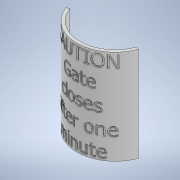
# Autodesk Inventor part: warningSignV1
Saved by Autodesk Inventor 2021.2 (Build 252289000, 289)
## iProperties
Created: 2020-11-24
Part Number: warningSignV1
Material: Generic
Document SubType Name: Modeling
Designer: robst
Density: 1 g/cm^3
Appearance: Default
Author: robst
Autodesk Inventor part; units mm, degrees
ref_plane "YZ Plane" through (0, 0, 0) normal (1, 0, 0) x (0, 1, 0)
ref_plane "XZ Plane" through (0, 0, 0) normal (0, 1, 0) x (-1, 0, 0)
sketch "Sketch1" plane through (0, 0, 0) normal (0, 1, 0) x (-1, 0, 0)
  arc A0 (65.9911, 38.1) -> (-65.4234, 39.0668) centre (0, 0) ccw
  arc A1 (72.6124, 39.2675) -> (-71.4904, 41.275) centre (0, 0) ccw
  line L0 (0, 0) -> (0, -82.55) construction
  arc A2 (71.6046, 26.0619) -> (-71.6046, 26.0619) centre (0, 0) ccw
  arc A3 (77.5716, 28.2338) -> (-77.5716, 28.2338) centre (0, 0) ccw
  line L1 (0, 0) -> (77.5716, 28.2338) construction
  line L2 (0, 0) -> (-77.5716, 28.2338) construction
  line L3 (-77.5716, 28.2338) -> (-71.6046, 26.0619)
  line L4 (77.5716, 28.2338) -> (71.6046, 26.0619)
  point P0 (-65.4234, 39.0668)
  point P1 (65.9911, 38.1)
  point P2 (72.6124, 39.2675)
  point P3 (-71.4904, 41.275)
  dimension "d0" = 152.4
  dimension "d9" = 6.35
  dimension "d10" = 110
  dimension "d11" = 110
  constraints: 10 end point, 8 point on circle, 4 centre point, 4 coincident, 2 concentric, 2 point on line, 1 vertical
  measures "d0" diameter of A0
  measures "d9" radial gap between concentric circles of A1 A0
  measures "d10" angle of L1 L0
  measures "d11" angle of L2 L0
extrude "Extrusion1" add sketch "Sketch1" along normal blind 203.2
ref_plane "Work Plane1" through (0, 0, 82.55) normal (0, 0, 1) x (1, 0, 0)
sketch "Sketch3" plane through (0, 0, 82.55) normal (0, 0, 1) x (1, 0, 0)
  line L0 (-72.043, 0) -> (-72.043, 203.2) projected
  line L1 (71.4904, 0) -> (71.4904, 203.2) projected
  line L2 (77.5716, 203.2) -> (-77.5716, 203.2) projected
  line L3 (77.5716, 0) -> (-77.5716, 0) projected
  line L4 (-72.043, 177.8) -> (71.4904, 177.8) construction
  spline S0 degree 2 poles (-60.9358, 172.2672) (-63.4058, 172.2672) (-67.5842, 173.9344) (-69.1074, 175.6017) knots 0 0 0 1 2 2 2
  spline S1 degree 2 poles (-69.1074, 175.6017) (-70.6306, 177.2484) (-72.2979, 182.1884) (-72.2979, 185.3994) knots 0 0 0 1 2 2 2
  spline S2 degree 2 poles (-72.2979, 185.3994) (-72.2979, 188.5899) (-70.6718, 193.3241) (-69.128, 195.0736) knots 0 0 0 1 2 2 2
  spline S3 degree 2 poles (-69.128, 195.0736) (-67.6048, 196.7821) (-63.447, 198.5728) (-60.874, 198.5728) knots 0 0 0 1 2 2 2
  spline S4 degree 2 poles (-60.874, 198.5728) (-59.5979, 198.5728) (-57.3543, 198.2023) (-56.4074, 197.9142) knots 0 0 0 1 2 2 2
  spline S5 degree 2 poles (-56.4074, 197.9142) (-55.5841, 197.6466) (-53.8757, 196.885) (-53.0317, 196.4322) knots 0 0 0 1 2 2 2
  line L5 (-53.0317, 196.4322) -> (-53.0317, 192.3566)
  line L6 (-53.0317, 192.3566) -> (-53.2993, 192.3566)
  spline S6 degree 2 poles (-53.2993, 192.3566) (-53.7522, 192.7683) (-55.1518, 193.921) (-56.1604, 194.4767) knots 0 0 0 1 2 2 2
  spline S7 degree 2 poles (-56.1604, 194.4767) (-57.1278, 195.0119) (-59.4126, 195.6912) (-60.8946, 195.6912) knots 0 0 0 1 2 2 2
  spline S8 degree 2 poles (-60.8946, 195.6912) (-62.5207, 195.6912) (-65.423, 194.3532) (-66.5139, 193.077) knots 0 0 0 1 2 2 2
  spline S9 degree 2 poles (-66.5139, 193.077) (-67.5842, 191.7803) (-68.7781, 187.8488) (-68.7781, 185.3994) knots 0 0 0 1 2 2 2
  spline S10 degree 2 poles (-68.7781, 185.3994) (-68.7781, 182.7853) (-67.5225, 179.0185) (-66.4316, 177.7218) knots 0 0 0 1 2 2 2
  spline S11 degree 2 poles (-66.4316, 177.7218) (-65.3612, 176.4662) (-62.5001, 175.19) (-60.8946, 175.19) knots 0 0 0 1 2 2 2
  spline S12 degree 2 poles (-60.8946, 175.19) (-59.4332, 175.19) (-56.9426, 175.9104) (-55.9752, 176.4456) knots 0 0 0 1 2 2 2
  spline S13 degree 2 poles (-55.9752, 176.4456) (-55.0489, 176.9808) (-53.6698, 178.0923) (-53.2787, 178.4834) knots 0 0 0 1 2 2 2
  line L7 (-53.2787, 178.4834) -> (-53.0317, 178.4834)
  line L8 (-53.0317, 178.4834) -> (-53.0317, 174.449)
  spline S14 degree 2 poles (-53.0317, 174.449) (-53.8757, 174.0579) (-55.3577, 173.3375) (-56.4074, 173.0082) knots 0 0 0 1 2 2 2
  spline S15 degree 2 poles (-56.4074, 173.0082) (-57.5189, 172.6377) (-59.4126, 172.2672) (-60.9358, 172.2672) knots 0 0 0 1 2 2 2
  line L9 (-52.6201, 172.72) -> (-44.0573, 198.12)
  line L10 (-44.0573, 198.12) -> (-39.8995, 198.12)
  line L11 (-39.8995, 198.12) -> (-31.3368, 172.72)
  line L12 (-31.3368, 172.72) -> (-34.8977, 172.72)
  line L13 (-34.8977, 172.72) -> (-37.203, 179.8213)
  line L14 (-37.203, 179.8213) -> (-46.8979, 179.8213)
  line L15 (-46.8979, 179.8213) -> (-49.2032, 172.72)
  line L16 (-49.2032, 172.72) -> (-52.6201, 172.72)
  line L17 (-38.1293, 182.703) -> (-42.0607, 194.662)
  line L18 (-42.0607, 194.662) -> (-45.9716, 182.703)
  line L19 (-45.9716, 182.703) -> (-38.1293, 182.703)
  spline S16 degree 2 poles (-19.7277, 172.1848) (-21.9713, 172.1848) (-25.3058, 173.3581) (-26.4791, 174.5313) knots 0 0 0 1 2 2 2
  spline S17 degree 2 poles (-26.4791, 174.5313) (-27.817, 175.8487) (-28.9079, 179.5537) (-28.9079, 182.2707) knots 0 0 0 1 2 2 2
  line L20 (-28.9079, 182.2707) -> (-28.9079, 198.12)
  line L21 (-28.9079, 198.12) -> (-25.5322, 198.12)
  line L22 (-25.5322, 198.12) -> (-25.5322, 182.2707)
  spline S18 degree 2 poles (-25.5322, 182.2707) (-25.5322, 180.5006) (-25.0794, 178.1129) (-24.4413, 177.1454) knots 0 0 0 1 2 2 2
  spline S19 degree 2 poles (-24.4413, 177.1454) (-23.762, 176.1163) (-21.4155, 175.0665) (-19.7277, 175.0665) knots 0 0 0 1 2 2 2
  spline S20 degree 2 poles (-19.7277, 175.0665) (-18.1428, 175.0665) (-15.6727, 176.1163) (-14.9935, 177.1454) knots 0 0 0 1 2 2 2
  spline S21 degree 2 poles (-14.9935, 177.1454) (-14.3554, 178.1129) (-13.9026, 180.48) (-13.9026, 182.1884) knots 0 0 0 1 2 2 2
  line L23 (-13.9026, 182.1884) -> (-13.9026, 198.12)
  line L24 (-13.9026, 198.12) -> (-10.5269, 198.12)
  line L25 (-10.5269, 198.12) -> (-10.5269, 182.2707)
  spline S22 degree 2 poles (-10.5269, 182.2707) (-10.5269, 179.6155) (-11.5972, 175.8281) (-12.9557, 174.5313) knots 0 0 0 1 2 2 2
  spline S23 degree 2 poles (-12.9557, 174.5313) (-14.1701, 173.3375) (-17.3812, 172.1848) (-19.7277, 172.1848) knots 0 0 0 1 2 2 2
  line L26 (0.2383, 172.72) -> (0.2383, 195.1148)
  line L27 (0.2383, 195.1148) -> (-8.2833, 195.1148)
  line L28 (-8.2833, 195.1148) -> (-8.2833, 198.12)
  line L29 (-8.2833, 198.12) -> (12.1355, 198.12)
  line L30 (12.1355, 198.12) -> (12.1355, 195.1148)
  line L31 (12.1355, 195.1148) -> (3.614, 195.1148)
  line L32 (3.614, 195.1148) -> (3.614, 172.72)
  line L33 (3.614, 172.72) -> (0.2383, 172.72)
  line L34 (23.5799, 172.72) -> (13.741, 172.72)
  line L35 (13.741, 172.72) -> (13.741, 175.3135)
  line L36 (13.741, 175.3135) -> (16.9726, 175.3135)
  line L37 (16.9726, 175.3135) -> (16.9726, 195.5265)
  line L38 (16.9726, 195.5265) -> (13.741, 195.5265)
  line L39 (13.741, 195.5265) -> (13.741, 198.12)
  line L40 (13.741, 198.12) -> (23.5799, 198.12)
  line L41 (23.5799, 198.12) -> (23.5799, 195.5265)
  line L42 (23.5799, 195.5265) -> (20.3483, 195.5265)
  line L43 (20.3483, 195.5265) -> (20.3483, 175.3135)
  line L44 (20.3483, 175.3135) -> (23.5799, 175.3135)
  line L45 (23.5799, 175.3135) -> (23.5799, 172.72)
  spline S24 degree 2 poles (45.7277, 195.2177) (47.1686, 193.5299) (48.7741, 188.5899) (48.7741, 185.42) knots 0 0 0 1 2 2 2
  spline S25 degree 2 poles (48.7741, 185.42) (48.7741, 182.3325) (47.2098, 177.3307) (45.7277, 175.6429) knots 0 0 0 1 2 2 2
  spline S26 degree 2 poles (45.7277, 175.6429) (44.1634, 173.8727) (40.0261, 172.1848) (37.5355, 172.1848) knots 0 0 0 1 2 2 2
  spline S27 degree 2 poles (37.5355, 172.1848) (34.9626, 172.1848) (30.8459, 173.9344) (29.3433, 175.6429) knots 0 0 0 1 2 2 2
  spline S28 degree 2 poles (29.3433, 175.6429) (27.8819, 177.3307) (26.3175, 182.2913) (26.3175, 185.42) knots 0 0 0 1 2 2 2
  spline S29 degree 2 poles (26.3175, 185.42) (26.3175, 188.6104) (27.9025, 193.4681) (29.3639, 195.2177) knots 0 0 0 1 2 2 2
  spline S30 degree 2 poles (29.3639, 195.2177) (30.8459, 196.9056) (34.9832, 198.6552) (37.5355, 198.6552) knots 0 0 0 1 2 2 2
  spline S31 degree 2 poles (37.5355, 198.6552) (40.129, 198.6552) (44.2869, 196.8438) (45.7277, 195.2177) knots 0 0 0 1 2 2 2
  spline S32 degree 2 poles (45.2543, 185.42) (45.2543, 187.9312) (44.1634, 191.8215) (43.1754, 193.0976) knots 0 0 0 1 2 2 2
  spline S33 degree 2 poles (43.1754, 193.0976) (42.1668, 194.415) (39.3263, 195.7323) (37.5561, 195.7323) knots 0 0 0 1 2 2 2
  spline S34 degree 2 poles (37.5561, 195.7323) (35.7242, 195.7323) (32.966, 194.4561) (31.9162, 193.0976) knots 0 0 0 1 2 2 2
  spline S35 degree 2 poles (31.9162, 193.0976) (30.9076, 191.8009) (29.8373, 187.89) (29.8373, 185.42) knots 0 0 0 1 2 2 2
  spline S36 degree 2 poles (29.8373, 185.42) (29.8373, 180.4182) (34.0363, 175.1077) (37.5561, 175.1077) knots 0 0 0 1 2 2 2
  spline S37 degree 2 poles (37.5561, 175.1077) (41.0759, 175.1077) (45.2543, 180.4182) (45.2543, 185.42) knots 0 0 0 1 2 2 2
  line L46 (70.6543, 172.72) -> (66.867, 172.72)
  line L47 (66.867, 172.72) -> (55.6284, 194.6208)
  line L48 (55.6284, 194.6208) -> (55.6284, 172.72)
  line L49 (55.6284, 172.72) -> (52.4791, 172.72)
  line L50 (52.4791, 172.72) -> (52.4791, 198.12)
  line L51 (52.4791, 198.12) -> (57.2751, 198.12)
  line L52 (57.2751, 198.12) -> (67.5051, 178.01)
  line L53 (67.5051, 178.01) -> (67.5051, 198.12)
  line L54 (67.5051, 198.12) -> (70.6543, 198.12)
  line L55 (70.6543, 198.12) -> (70.6543, 172.72)
  spline S38 degree 2 poles (-22.9284, 130.3638) (-25.6248, 130.3638) (-30.0915, 132.0105) (-31.697, 133.6777) knots 0 0 0 1 2 2 2
  spline S39 degree 2 poles (-31.697, 133.6777) (-33.3025, 135.3656) (-35.0109, 140.3468) (-35.0109, 143.5784) knots 0 0 0 1 2 2 2
  spline S40 degree 2 poles (-35.0109, 143.5784) (-35.0109, 146.6453) (-33.2819, 151.503) (-31.6764, 153.232) knots 0 0 0 1 2 2 2
  spline S41 degree 2 poles (-31.6764, 153.232) (-30.1326, 154.8993) (-25.6043, 156.7106) (-22.9078, 156.7106) knots 0 0 0 1 2 2 2
  spline S42 degree 2 poles (-22.9078, 156.7106) (-21.6111, 156.7106) (-19.2646, 156.3401) (-18.1942, 156.0108) knots 0 0 0 1 2 2 2
  spline S43 degree 2 poles (-18.1942, 156.0108) (-17.3297, 155.7638) (-15.2302, 154.8581) (-14.5921, 154.5288) knots 0 0 0 1 2 2 2
  line L56 (-14.5921, 154.5288) -> (-14.5921, 150.4533)
  line L57 (-14.5921, 150.4533) -> (-14.8803, 150.4533)
  spline S44 degree 2 poles (-14.8803, 150.4533) (-15.5184, 151.009) (-16.8563, 152.0176) (-18.0913, 152.594) knots 0 0 0 1 2 2 2
  spline S45 degree 2 poles (-18.0913, 152.594) (-19.1205, 153.1085) (-21.7757, 153.7878) (-23.2989, 153.7878) knots 0 0 0 1 2 2 2
  spline S46 degree 2 poles (-23.2989, 153.7878) (-26.9628, 153.7878) (-31.4911, 148.2714) (-31.4911, 143.6813) knots 0 0 0 1 2 2 2
  spline S47 degree 2 poles (-31.4911, 143.6813) (-31.4911, 141.129) (-30.2973, 137.3004) (-29.1652, 135.9831) knots 0 0 0 1 2 2 2
  spline S48 degree 2 poles (-29.1652, 135.9831) (-28.0743, 134.6658) (-24.9868, 133.2867) (-23.0519, 133.2867) knots 0 0 0 1 2 2 2
  spline S49 degree 2 poles (-23.0519, 133.2867) (-21.6317, 133.2867) (-18.7911, 133.6983) (-17.8237, 134.11) knots 0 0 0 1 2 2 2
  line L58 (-17.8237, 134.11) -> (-17.8237, 140.6761)
  line L59 (-17.8237, 140.6761) -> (-23.7106, 140.6761)
  line L60 (-23.7106, 140.6761) -> (-23.7106, 143.6401)
  line L61 (-23.7106, 143.6401) -> (-14.4892, 143.6401)
  line L62 (-14.4892, 143.6401) -> (-14.4892, 132.5457)
  spline S50 degree 2 poles (-14.4892, 132.5457) (-15.1273, 132.2575) (-17.3091, 131.3724) (-18.2354, 131.1048) knots 0 0 0 1 2 2 2
  spline S51 degree 2 poles (-18.2354, 131.1048) (-19.491, 130.7343) (-21.5082, 130.3638) (-22.9284, 130.3638) knots 0 0 0 1 2 2 2
  spline S52 degree 2 poles (0.1251, 132.875) (-0.266, 132.5868) (-1.5834, 131.5576) (-2.2009, 131.2489) knots 0 0 0 1 2 2 2
  spline S53 degree 2 poles (-2.2009, 131.2489) (-3.0448, 130.7961) (-4.6297, 130.3226) (-6.0706, 130.3226) knots 0 0 0 1 2 2 2
  spline S54 degree 2 poles (-6.0706, 130.3226) (-7.2438, 130.3226) (-9.3639, 131.2077) (-10.1667, 132.0105) knots 0 0 0 1 2 2 2
  spline S55 degree 2 poles (-10.1667, 132.0105) (-10.9282, 132.7927) (-11.8545, 135.098) (-11.8545, 136.3742) knots 0 0 0 1 2 2 2
  spline S56 degree 2 poles (-11.8545, 136.3742) (-11.8545, 138.3502) (-10.1872, 141.1495) (-8.3759, 141.9523) knots 0 0 0 1 2 2 2
  spline S57 degree 2 poles (-8.3759, 141.9523) (-6.7704, 142.6933) (-2.4067, 143.2491) (0.1251, 143.3931) knots 0 0 0 1 2 2 2
  line L63 (0.1251, 143.3931) -> (0.1251, 144.0106)
  spline S58 degree 2 poles (0.1251, 144.0106) (0.1251, 145.1222) (-0.5542, 146.5012) (-1.1717, 146.8923) knots 0 0 0 1 2 2 2
  spline S59 degree 2 poles (-1.1717, 146.8923) (-1.7892, 147.2834) (-3.5594, 147.5304) (-4.5062, 147.5304) knots 0 0 0 1 2 2 2
  spline S60 degree 2 poles (-4.5062, 147.5304) (-5.6177, 147.5304) (-8.6229, 146.8717) (-10.1255, 146.2337) knots 0 0 0 1 2 2 2
  line L64 (-10.1255, 146.2337) -> (-10.3107, 146.2337)
  line L65 (-10.3107, 146.2337) -> (-10.3107, 149.5064)
  spline S61 degree 2 poles (-10.3107, 149.5064) (-9.4257, 149.7534) (-6.1117, 150.3709) (-4.4856, 150.3709) knots 0 0 0 1 2 2 2
  spline S62 degree 2 poles (-4.4856, 150.3709) (-2.5096, 150.3709) (0.1868, 149.7534) (1.2572, 148.9507) knots 0 0 0 1 2 2 2
  spline S63 degree 2 poles (1.2572, 148.9507) (2.3069, 148.1685) (3.3361, 145.6779) (3.3361, 143.8871) knots 0 0 0 1 2 2 2
  line L66 (3.3361, 143.8871) -> (3.3361, 130.8578)
  line L67 (3.3361, 130.8578) -> (0.1251, 130.8578)
  line L68 (0.1251, 130.8578) -> (0.1251, 132.875)
  line L69 (0.1251, 135.5508) -> (0.1251, 140.8408)
  spline S64 degree 2 poles (0.1251, 140.8408) (-1.0276, 140.7379) (-4.5062, 140.388) (-5.5971, 140.0586) knots 0 0 0 1 2 2 2
  spline S65 degree 2 poles (-5.5971, 140.0586) (-6.8733, 139.6675) (-8.5406, 138.0414) (-8.5406, 136.6006) knots 0 0 0 1 2 2 2
  spline S66 degree 2 poles (-8.5406, 136.6006) (-8.5406, 134.9539) (-6.6881, 133.2867) (-4.9179, 133.2867) knots 0 0 0 1 2 2 2
  spline S67 degree 2 poles (-4.9179, 133.2867) (-3.4153, 133.2867) (-0.9453, 134.5834) (0.1251, 135.5508) knots 0 0 0 1 2 2 2
  spline S68 degree 2 poles (13.6072, 130.4873) (10.9931, 130.4873) (8.0497, 133.4719) (8.0497, 136.7035) knots 0 0 0 1 2 2 2
  line L70 (8.0497, 136.7035) -> (8.0497, 147.2628)
  line L71 (8.0497, 147.2628) -> (5.8884, 147.2628)
  line L72 (5.8884, 147.2628) -> (5.8884, 149.9181)
  line L73 (5.8884, 149.9181) -> (8.0497, 149.9181)
  line L74 (8.0497, 149.9181) -> (8.0497, 155.3933)
  line L75 (8.0497, 155.3933) -> (11.2607, 155.3933)
  line L76 (11.2607, 155.3933) -> (11.2607, 149.9181)
  line L77 (11.2607, 149.9181) -> (17.1682, 149.9181)
  line L78 (17.1682, 149.9181) -> (17.1682, 147.2628)
  line L79 (17.1682, 147.2628) -> (11.2607, 147.2628)
  line L80 (11.2607, 147.2628) -> (11.2607, 138.1855)
  spline S69 degree 2 poles (11.2607, 138.1855) (11.2607, 136.7447) (11.3636, 135.1598) (11.7136, 134.4805) knots 0 0 0 1 2 2 2
  spline S70 degree 2 poles (11.7136, 134.4805) (12.0017, 133.8836) (13.2985, 133.2867) (14.41, 133.2867) knots 0 0 0 1 2 2 2
  spline S71 degree 2 poles (14.41, 133.2867) (15.1922, 133.2867) (16.6536, 133.7601) (16.9829, 133.9042) knots 0 0 0 1 2 2 2
  line L81 (16.9829, 133.9042) -> (17.1682, 133.9042)
  line L82 (17.1682, 133.9042) -> (17.1682, 131.0225)
  spline S72 degree 2 poles (17.1682, 131.0225) (16.2625, 130.7755) (14.41, 130.4873) (13.6072, 130.4873) knots 0 0 0 1 2 2 2
  spline S73 degree 2 poles (27.8098, 130.4256) (23.2403, 130.4256) (18.2179, 135.5508) (18.2179, 140.285) knots 0 0 0 1 2 2 2
  spline S74 degree 2 poles (18.2179, 140.285) (18.2179, 144.9369) (23.0962, 150.4533) (27.0277, 150.4533) knots 0 0 0 1 2 2 2
  spline S75 degree 2 poles (27.0277, 150.4533) (28.7978, 150.4533) (31.5354, 149.4241) (32.544, 148.3332) knots 0 0 0 1 2 2 2
  spline S76 degree 2 poles (32.544, 148.3332) (33.5732, 147.2423) (34.6641, 144.093) (34.6641, 141.8082) knots 0 0 0 1 2 2 2
  line L83 (34.6641, 141.8082) -> (34.6641, 140.0586)
  line L84 (34.6641, 140.0586) -> (21.4701, 140.0586)
  spline S77 degree 2 poles (21.4701, 140.0586) (21.4701, 136.7447) (24.8047, 133.2249) (27.7687, 133.2249) knots 0 0 0 1 2 2 2
  spline S78 degree 2 poles (27.7687, 133.2249) (28.8184, 133.2249) (30.8562, 133.6983) (31.6795, 134.0688) knots 0 0 0 1 2 2 2
  spline S79 degree 2 poles (31.6795, 134.0688) (32.544, 134.4805) (33.7379, 135.2009) (34.129, 135.5303) knots 0 0 0 1 2 2 2
  line L85 (34.129, 135.5303) -> (34.3142, 135.5303)
  line L86 (34.3142, 135.5303) -> (34.3142, 132.0311)
  spline S80 degree 2 poles (34.3142, 132.0311) (33.7585, 131.8046) (32.0706, 131.146) (31.4119, 130.9607) knots 0 0 0 1 2 2 2
  spline S81 degree 2 poles (31.4119, 130.9607) (30.4857, 130.6931) (28.9625, 130.4256) (27.8098, 130.4256) knots 0 0 0 1 2 2 2
  spline S82 degree 2 poles (31.5354, 142.5081) (31.4943, 143.8048) (30.9591, 145.6985) (30.4445, 146.3366) knots 0 0 0 1 2 2 2
  spline S83 degree 2 poles (30.4445, 146.3366) (29.8888, 147.057) (28.1392, 147.8186) (26.8424, 147.8186) knots 0 0 0 1 2 2 2
  spline S84 degree 2 poles (26.8424, 147.8186) (25.5662, 147.8186) (23.7755, 147.057) (23.0345, 146.316) knots 0 0 0 1 2 2 2
  spline S85 degree 2 poles (23.0345, 146.316) (22.3141, 145.5544) (21.573, 143.7225) (21.4701, 142.5081) knots 0 0 0 1 2 2 2
  line L87 (21.4701, 142.5081) -> (31.5354, 142.5081)
  spline S86 degree 2 poles (-36.6782, 87.8841) (-38.6542, 87.8841) (-41.927, 89.0985) (-43.1002, 90.3335) knots 0 0 0 1 2 2 2
  spline S87 degree 2 poles (-43.1002, 90.3335) (-44.2735, 91.548) (-45.5702, 95.2942) (-45.5702, 97.8053) knots 0 0 0 1 2 2 2
  spline S88 degree 2 poles (-45.5702, 97.8053) (-45.5702, 100.3165) (-44.2323, 103.9804) (-43.1002, 105.2154) knots 0 0 0 1 2 2 2
  spline S89 degree 2 poles (-43.1002, 105.2154) (-41.9681, 106.471) (-38.613, 107.8089) (-36.6782, 107.8089) knots 0 0 0 1 2 2 2
  spline S90 degree 2 poles (-36.6782, 107.8089) (-35.1138, 107.8089) (-32.191, 106.9238) (-31.0589, 106.3475) knots 0 0 0 1 2 2 2
  line L88 (-31.0589, 106.3475) -> (-31.0589, 102.7454)
  line L89 (-31.0589, 102.7454) -> (-31.2441, 102.7454)
  spline S91 degree 2 poles (-31.2441, 102.7454) (-31.594, 103.0335) (-32.6644, 103.7746) (-33.426, 104.1656) knots 0 0 0 1 2 2 2
  spline S92 degree 2 poles (-33.426, 104.1656) (-34.1052, 104.495) (-35.9166, 105.0096) (-36.7399, 105.0096) knots 0 0 0 1 2 2 2
  spline S93 degree 2 poles (-36.7399, 105.0096) (-39.2305, 105.0096) (-42.2563, 101.2428) (-42.2563, 97.8053) knots 0 0 0 1 2 2 2
  spline S94 degree 2 poles (-42.2563, 97.8053) (-42.2563, 94.4502) (-39.3334, 90.6835) (-36.7399, 90.6835) knots 0 0 0 1 2 2 2
  spline S95 degree 2 poles (-36.7399, 90.6835) (-35.1756, 90.6835) (-32.3351, 91.9802) (-31.2441, 92.9888) knots 0 0 0 1 2 2 2
  line L90 (-31.2441, 92.9888) -> (-31.0589, 92.9888)
  line L91 (-31.0589, 92.9888) -> (-31.0589, 89.3867)
  spline S96 degree 2 poles (-31.0589, 89.3867) (-31.5323, 89.1603) (-32.9731, 88.5222) (-33.5495, 88.3781) knots 0 0 0 1 2 2 2
  spline S97 degree 2 poles (-33.5495, 88.3781) (-34.3728, 88.1311) (-35.6696, 87.8841) (-36.6782, 87.8841) knots 0 0 0 1 2 2 2
  line L92 (-24.8633, 88.3164) -> (-28.0743, 88.3164)
  line L93 (-28.0743, 88.3164) -> (-28.0743, 114.8485)
  line L94 (-28.0743, 114.8485) -> (-24.8633, 114.8485)
  line L95 (-24.8633, 114.8485) -> (-24.8633, 88.3164)
  spline S98 degree 2 poles (-4.4856, 97.8465) (-4.4856, 93.03) (-9.1169, 87.7812) (-12.9866, 87.7812) knots 0 0 0 1 2 2 2
  spline S99 degree 2 poles (-12.9866, 87.7812) (-16.9592, 87.7812) (-21.5082, 93.1946) (-21.5082, 97.8465) knots 0 0 0 1 2 2 2
  spline S100 degree 2 poles (-21.5082, 97.8465) (-21.5082, 102.6219) (-16.8151, 107.9118) (-12.9866, 107.9118) knots 0 0 0 1 2 2 2
  spline S101 degree 2 poles (-12.9866, 107.9118) (-9.1169, 107.9118) (-4.4856, 102.6425) (-4.4856, 97.8465) knots 0 0 0 1 2 2 2
  spline S102 degree 2 poles (-7.7996, 97.8465) (-7.7996, 101.5515) (-10.496, 105.1536) (-12.9866, 105.1536) knots 0 0 0 1 2 2 2
  spline S103 degree 2 poles (-12.9866, 105.1536) (-15.4772, 105.1536) (-18.1942, 101.5515) (-18.1942, 97.8465) knots 0 0 0 1 2 2 2
  spline S104 degree 2 poles (-18.1942, 97.8465) (-18.1942, 94.2444) (-15.4772, 90.5394) (-12.9866, 90.5394) knots 0 0 0 1 2 2 2
  spline S105 degree 2 poles (-12.9866, 90.5394) (-10.5166, 90.5394) (-7.7996, 94.1827) (-7.7996, 97.8465) knots 0 0 0 1 2 2 2
  spline S106 degree 2 poles (3.9536, 87.8635) (2.0393, 87.8635) (-1.2746, 88.8927) (-2.3655, 89.469) knots 0 0 0 1 2 2 2
  line L96 (-2.3655, 89.469) -> (-2.3655, 93.0711)
  line L97 (-2.3655, 93.0711) -> (-2.2009, 93.0711)
  spline S107 degree 2 poles (-2.2009, 93.0711) (-1.7892, 92.7418) (-0.6777, 91.9596) (0.2486, 91.5274) knots 0 0 0 1 2 2 2
  spline S108 degree 2 poles (0.2486, 91.5274) (1.0513, 91.1363) (3.0273, 90.56) (4.0771, 90.56) knots 0 0 0 1 2 2 2
  spline S109 degree 2 poles (4.0771, 90.56) (4.8387, 90.56) (6.5883, 90.9099) (7, 91.1981) knots 0 0 0 1 2 2 2
  spline S110 degree 2 poles (7, 91.1981) (7.5969, 91.5891) (8.132, 92.4742) (8.132, 93.3799) knots 0 0 0 1 2 2 2
  spline S111 degree 2 poles (8.132, 93.3799) (8.132, 94.512) (6.897, 95.6852) (5.3121, 96.0763) knots 0 0 0 1 2 2 2
  spline S112 degree 2 poles (5.3121, 96.0763) (4.6946, 96.2204) (2.7186, 96.6321) (1.8747, 96.8585) knots 0 0 0 1 2 2 2
  spline S113 degree 2 poles (1.8747, 96.8585) (-0.3072, 97.4966) (-2.2832, 100.1313) (-2.2832, 102.0044) knots 0 0 0 1 2 2 2
  spline S114 degree 2 poles (-2.2832, 102.0044) (-2.2832, 104.5979) (1.6071, 107.8295) (4.8181, 107.8295) knots 0 0 0 1 2 2 2
  spline S115 degree 2 poles (4.8181, 107.8295) (6.403, 107.8295) (9.6141, 107.0473) (10.705, 106.4504) knots 0 0 0 1 2 2 2
  line L98 (10.705, 106.4504) -> (10.705, 103.013)
  line L99 (10.705, 103.013) -> (10.5403, 103.013)
  spline S116 degree 2 poles (10.5403, 103.013) (9.3053, 104.001) (6.3001, 105.1331) (4.7564, 105.1331) knots 0 0 0 1 2 2 2
  spline S117 degree 2 poles (4.7564, 105.1331) (3.1714, 105.1331) (0.9896, 103.7951) (0.9896, 102.4572) knots 0 0 0 1 2 2 2
  spline S118 degree 2 poles (0.9896, 102.4572) (0.9896, 101.2428) (2.2863, 100.0695) (3.7272, 99.699) knots 0 0 0 1 2 2 2
  spline S119 degree 2 poles (3.7272, 99.699) (4.427, 99.5138) (6.1972, 99.1433) (7.1646, 98.9169) knots 0 0 0 1 2 2 2
  spline S120 degree 2 poles (7.1646, 98.9169) (9.2641, 98.3817) (11.4048, 95.9322) (11.4048, 93.8122) knots 0 0 0 1 2 2 2
  spline S121 degree 2 poles (11.4048, 93.8122) (11.4048, 92.5771) (10.4374, 90.3953) (9.4906, 89.5925) knots 0 0 0 1 2 2 2
  spline S122 degree 2 poles (9.4906, 89.5925) (8.482, 88.7486) (5.909, 87.8635) (3.9536, 87.8635) knots 0 0 0 1 2 2 2
  spline S123 degree 2 poles (22.664, 87.8841) (18.0944, 87.8841) (13.0721, 93.0094) (13.0721, 97.7436) knots 0 0 0 1 2 2 2
  spline S124 degree 2 poles (13.0721, 97.7436) (13.0721, 102.3955) (17.9504, 107.9118) (21.8818, 107.9118) knots 0 0 0 1 2 2 2
  spline S125 degree 2 poles (21.8818, 107.9118) (23.652, 107.9118) (26.3896, 106.8827) (27.3982, 105.7917) knots 0 0 0 1 2 2 2
  spline S126 degree 2 poles (27.3982, 105.7917) (28.4273, 104.7008) (29.5183, 101.5515) (29.5183, 99.2668) knots 0 0 0 1 2 2 2
  line L100 (29.5183, 99.2668) -> (29.5183, 97.5172)
  line L101 (29.5183, 97.5172) -> (16.3243, 97.5172)
  spline S127 degree 2 poles (16.3243, 97.5172) (16.3243, 94.2032) (19.6588, 90.6835) (22.6228, 90.6835) knots 0 0 0 1 2 2 2
  spline S128 degree 2 poles (22.6228, 90.6835) (23.6726, 90.6835) (25.7103, 91.1569) (26.5337, 91.5274) knots 0 0 0 1 2 2 2
  spline S129 degree 2 poles (26.5337, 91.5274) (27.3982, 91.9391) (28.592, 92.6595) (28.9831, 92.9888) knots 0 0 0 1 2 2 2
  line L102 (28.9831, 92.9888) -> (29.1683, 92.9888)
  line L103 (29.1683, 92.9888) -> (29.1683, 89.4896)
  spline S130 degree 2 poles (29.1683, 89.4896) (28.6126, 89.2632) (26.9247, 88.6045) (26.2661, 88.4193) knots 0 0 0 1 2 2 2
  spline S131 degree 2 poles (26.2661, 88.4193) (25.3398, 88.1517) (23.8166, 87.8841) (22.664, 87.8841) knots 0 0 0 1 2 2 2
  spline S132 degree 2 poles (26.3896, 99.9666) (26.3484, 101.2634) (25.8132, 103.157) (25.2987, 103.7951) knots 0 0 0 1 2 2 2
  spline S133 degree 2 poles (25.2987, 103.7951) (24.7429, 104.5156) (22.9933, 105.2771) (21.6965, 105.2771) knots 0 0 0 1 2 2 2
  spline S134 degree 2 poles (21.6965, 105.2771) (20.4204, 105.2771) (18.6296, 104.5156) (17.8886, 103.7746) knots 0 0 0 1 2 2 2
  spline S135 degree 2 poles (17.8886, 103.7746) (17.1682, 103.013) (16.4272, 101.181) (16.3243, 99.9666) knots 0 0 0 1 2 2 2
  line L104 (16.3243, 99.9666) -> (26.3896, 99.9666)
  spline S136 degree 2 poles (37.9163, 87.8635) (36.0021, 87.8635) (32.6881, 88.8927) (31.5972, 89.469) knots 0 0 0 1 2 2 2
  line L105 (31.5972, 89.469) -> (31.5972, 93.0711)
  line L106 (31.5972, 93.0711) -> (31.7619, 93.0711)
  spline S137 degree 2 poles (31.7619, 93.0711) (32.1735, 92.7418) (33.285, 91.9596) (34.2113, 91.5274) knots 0 0 0 1 2 2 2
  spline S138 degree 2 poles (34.2113, 91.5274) (35.0141, 91.1363) (36.9901, 90.56) (38.0398, 90.56) knots 0 0 0 1 2 2 2
  spline S139 degree 2 poles (38.0398, 90.56) (38.8014, 90.56) (40.551, 90.9099) (40.9627, 91.1981) knots 0 0 0 1 2 2 2
  spline S140 degree 2 poles (40.9627, 91.1981) (41.5596, 91.5891) (42.0948, 92.4742) (42.0948, 93.3799) knots 0 0 0 1 2 2 2
  spline S141 degree 2 poles (42.0948, 93.3799) (42.0948, 94.512) (40.8598, 95.6852) (39.2748, 96.0763) knots 0 0 0 1 2 2 2
  spline S142 degree 2 poles (39.2748, 96.0763) (38.6573, 96.2204) (36.6813, 96.6321) (35.8374, 96.8585) knots 0 0 0 1 2 2 2
  spline S143 degree 2 poles (35.8374, 96.8585) (33.6555, 97.4966) (31.6795, 100.1313) (31.6795, 102.0044) knots 0 0 0 1 2 2 2
  spline S144 degree 2 poles (31.6795, 102.0044) (31.6795, 104.5979) (35.5698, 107.8295) (38.7808, 107.8295) knots 0 0 0 1 2 2 2
  spline S145 degree 2 poles (38.7808, 107.8295) (40.3658, 107.8295) (43.5768, 107.0473) (44.6677, 106.4504) knots 0 0 0 1 2 2 2
  line L107 (44.6677, 106.4504) -> (44.6677, 103.013)
  line L108 (44.6677, 103.013) -> (44.503, 103.013)
  spline S146 degree 2 poles (44.503, 103.013) (43.268, 104.001) (40.2628, 105.1331) (38.7191, 105.1331) knots 0 0 0 1 2 2 2
  spline S147 degree 2 poles (38.7191, 105.1331) (37.1341, 105.1331) (34.9523, 103.7951) (34.9523, 102.4572) knots 0 0 0 1 2 2 2
  spline S148 degree 2 poles (34.9523, 102.4572) (34.9523, 101.2428) (36.2491, 100.0695) (37.6899, 99.699) knots 0 0 0 1 2 2 2
  spline S149 degree 2 poles (37.6899, 99.699) (38.3897, 99.5138) (40.1599, 99.1433) (41.1273, 98.9169) knots 0 0 0 1 2 2 2
  spline S150 degree 2 poles (41.1273, 98.9169) (43.2269, 98.3817) (45.3675, 95.9322) (45.3675, 93.8122) knots 0 0 0 1 2 2 2
  spline S151 degree 2 poles (45.3675, 93.8122) (45.3675, 92.5771) (44.4001, 90.3953) (43.4533, 89.5925) knots 0 0 0 1 2 2 2
  spline S152 degree 2 poles (43.4533, 89.5925) (42.4447, 88.7486) (39.8718, 87.8635) (37.9163, 87.8635) knots 0 0 0 1 2 2 2
  spline S153 degree 2 poles (-57.2513, 47.6274) (-57.6424, 47.3393) (-58.9598, 46.3101) (-59.5773, 46.0013) knots 0 0 0 1 2 2 2
  spline S154 degree 2 poles (-59.5773, 46.0013) (-60.4212, 45.5485) (-62.0061, 45.0751) (-63.447, 45.0751) knots 0 0 0 1 2 2 2
  spline S155 degree 2 poles (-63.447, 45.0751) (-64.6202, 45.0751) (-66.7403, 45.9602) (-67.5431, 46.7629) knots 0 0 0 1 2 2 2
  spline S156 degree 2 poles (-67.5431, 46.7629) (-68.3047, 47.5451) (-69.2309, 49.8504) (-69.2309, 51.1266) knots 0 0 0 1 2 2 2
  spline S157 degree 2 poles (-69.2309, 51.1266) (-69.2309, 53.1026) (-67.5637, 55.902) (-65.7523, 56.7047) knots 0 0 0 1 2 2 2
  spline S158 degree 2 poles (-65.7523, 56.7047) (-64.1468, 57.4457) (-59.7831, 58.0015) (-57.2513, 58.1456) knots 0 0 0 1 2 2 2
  line L109 (-57.2513, 58.1456) -> (-57.2513, 58.7631)
  spline S159 degree 2 poles (-57.2513, 58.7631) (-57.2513, 59.8746) (-57.9306, 61.2537) (-58.5481, 61.6448) knots 0 0 0 1 2 2 2
  spline S160 degree 2 poles (-58.5481, 61.6448) (-59.1656, 62.0359) (-60.9358, 62.2829) (-61.8826, 62.2829) knots 0 0 0 1 2 2 2
  spline S161 degree 2 poles (-61.8826, 62.2829) (-62.9941, 62.2829) (-65.9993, 61.6242) (-67.5019, 60.9861) knots 0 0 0 1 2 2 2
  line L110 (-67.5019, 60.9861) -> (-67.6872, 60.9861)
  line L111 (-67.6872, 60.9861) -> (-67.6872, 64.2589)
  spline S162 degree 2 poles (-67.6872, 64.2589) (-66.8021, 64.5059) (-63.4881, 65.1234) (-61.862, 65.1234) knots 0 0 0 1 2 2 2
  spline S163 degree 2 poles (-61.862, 65.1234) (-59.886, 65.1234) (-57.1896, 64.5059) (-56.1192, 63.7031) knots 0 0 0 1 2 2 2
  spline S164 degree 2 poles (-56.1192, 63.7031) (-55.0695, 62.9209) (-54.0403, 60.4304) (-54.0403, 58.6396) knots 0 0 0 1 2 2 2
  line L112 (-54.0403, 58.6396) -> (-54.0403, 45.6103)
  line L113 (-54.0403, 45.6103) -> (-57.2513, 45.6103)
  line L114 (-57.2513, 45.6103) -> (-57.2513, 47.6274)
  line L115 (-57.2513, 50.3033) -> (-57.2513, 55.5932)
  spline S165 degree 2 poles (-57.2513, 55.5932) (-58.404, 55.4903) (-61.8826, 55.1404) (-62.9735, 54.8111) knots 0 0 0 1 2 2 2
  spline S166 degree 2 poles (-62.9735, 54.8111) (-64.2497, 54.42) (-65.917, 52.7939) (-65.917, 51.353) knots 0 0 0 1 2 2 2
  spline S167 degree 2 poles (-65.917, 51.353) (-65.917, 49.7064) (-64.0645, 48.0391) (-62.2943, 48.0391) knots 0 0 0 1 2 2 2
  spline S168 degree 2 poles (-62.2943, 48.0391) (-60.7917, 48.0391) (-58.3217, 49.3359) (-57.2513, 50.3033) knots 0 0 0 1 2 2 2
  line L116 (-39.5084, 69.0548) -> (-39.6731, 69.0548)
  spline S169 degree 2 poles (-39.6731, 69.0548) (-40.1053, 69.2195) (-41.7108, 69.5077) (-42.3489, 69.5077) knots 0 0 0 1 2 2 2
  spline S170 degree 2 poles (-42.3489, 69.5077) (-44.3661, 69.5077) (-46.0951, 67.6963) (-46.0951, 65.3086) knots 0 0 0 1 2 2 2
  line L117 (-46.0951, 65.3086) -> (-46.0951, 64.6705)
  line L118 (-46.0951, 64.6705) -> (-40.7846, 64.6705)
  line L119 (-40.7846, 64.6705) -> (-40.7846, 62.0153)
  line L120 (-40.7846, 62.0153) -> (-45.9922, 62.0153)
  line L121 (-45.9922, 62.0153) -> (-45.9922, 45.6103)
  line L122 (-45.9922, 45.6103) -> (-49.2032, 45.6103)
  line L123 (-49.2032, 45.6103) -> (-49.2032, 62.0153)
  line L124 (-49.2032, 62.0153) -> (-51.3645, 62.0153)
  line L125 (-51.3645, 62.0153) -> (-51.3645, 64.6705)
  line L126 (-51.3645, 64.6705) -> (-49.2032, 64.6705)
  line L127 (-49.2032, 64.6705) -> (-49.2032, 65.3086)
  spline S171 degree 2 poles (-49.2032, 65.3086) (-49.2032, 68.7255) (-45.8893, 72.307) (-42.8017, 72.307) knots 0 0 0 1 2 2 2
  spline S172 degree 2 poles (-42.8017, 72.307) (-41.9167, 72.307) (-40.2082, 72.1218) (-39.5084, 71.9983) knots 0 0 0 1 2 2 2
  line L128 (-39.5084, 71.9983) -> (-39.5084, 69.0548)
  spline S173 degree 2 poles (-31.9131, 45.2398) (-34.5272, 45.2398) (-37.4706, 48.2244) (-37.4706, 51.456) knots 0 0 0 1 2 2 2
  line L129 (-37.4706, 51.456) -> (-37.4706, 62.0153)
  line L130 (-37.4706, 62.0153) -> (-39.6319, 62.0153)
  line L131 (-39.6319, 62.0153) -> (-39.6319, 64.6705)
  line L132 (-39.6319, 64.6705) -> (-37.4706, 64.6705)
  line L133 (-37.4706, 64.6705) -> (-37.4706, 70.1457)
  line L134 (-37.4706, 70.1457) -> (-34.2596, 70.1457)
  line L135 (-34.2596, 70.1457) -> (-34.2596, 64.6705)
  line L136 (-34.2596, 64.6705) -> (-28.3522, 64.6705)
  line L137 (-28.3522, 64.6705) -> (-28.3522, 62.0153)
  line L138 (-28.3522, 62.0153) -> (-34.2596, 62.0153)
  line L139 (-34.2596, 62.0153) -> (-34.2596, 52.938)
  spline S174 degree 2 poles (-34.2596, 52.938) (-34.2596, 51.4971) (-34.1567, 49.9122) (-33.8068, 49.2329) knots 0 0 0 1 2 2 2
  spline S175 degree 2 poles (-33.8068, 49.2329) (-33.5186, 48.636) (-32.2218, 48.0391) (-31.1103, 48.0391) knots 0 0 0 1 2 2 2
  spline S176 degree 2 poles (-31.1103, 48.0391) (-30.3282, 48.0391) (-28.8667, 48.5125) (-28.5374, 48.6566) knots 0 0 0 1 2 2 2
  line L140 (-28.5374, 48.6566) -> (-28.3522, 48.6566)
  line L141 (-28.3522, 48.6566) -> (-28.3522, 45.7749)
  spline S177 degree 2 poles (-28.3522, 45.7749) (-29.2578, 45.5279) (-31.1103, 45.2398) (-31.9131, 45.2398) knots 0 0 0 1 2 2 2
  spline S178 degree 2 poles (-17.7105, 45.178) (-22.28, 45.178) (-27.3024, 50.3033) (-27.3024, 55.0375) knots 0 0 0 1 2 2 2
  spline S179 degree 2 poles (-27.3024, 55.0375) (-27.3024, 59.6893) (-22.4241, 65.2057) (-18.4927, 65.2057) knots 0 0 0 1 2 2 2
  spline S180 degree 2 poles (-18.4927, 65.2057) (-16.7225, 65.2057) (-13.9849, 64.1765) (-12.9763, 63.0856) knots 0 0 0 1 2 2 2
  spline S181 degree 2 poles (-12.9763, 63.0856) (-11.9471, 61.9947) (-10.8562, 58.8454) (-10.8562, 56.5607) knots 0 0 0 1 2 2 2
  line L142 (-10.8562, 56.5607) -> (-10.8562, 54.8111)
  line L143 (-10.8562, 54.8111) -> (-24.0502, 54.8111)
  spline S182 degree 2 poles (-24.0502, 54.8111) (-24.0502, 51.4971) (-20.7157, 47.9774) (-17.7517, 47.9774) knots 0 0 0 1 2 2 2
  spline S183 degree 2 poles (-17.7517, 47.9774) (-16.7019, 47.9774) (-14.6641, 48.4508) (-13.8408, 48.8213) knots 0 0 0 1 2 2 2
  spline S184 degree 2 poles (-13.8408, 48.8213) (-12.9763, 49.2329) (-11.7825, 49.9534) (-11.3914, 50.2827) knots 0 0 0 1 2 2 2
  line L144 (-11.3914, 50.2827) -> (-11.2061, 50.2827)
  line L145 (-11.2061, 50.2827) -> (-11.2061, 46.7835)
  spline S185 degree 2 poles (-11.2061, 46.7835) (-11.7619, 46.5571) (-13.4497, 45.8984) (-14.1084, 45.7132) knots 0 0 0 1 2 2 2
  spline S186 degree 2 poles (-14.1084, 45.7132) (-15.0346, 45.4456) (-16.5578, 45.178) (-17.7105, 45.178) knots 0 0 0 1 2 2 2
  spline S187 degree 2 poles (-13.9849, 57.2605) (-14.0261, 58.5573) (-14.5612, 60.4509) (-15.0758, 61.089) knots 0 0 0 1 2 2 2
  spline S188 degree 2 poles (-15.0758, 61.089) (-15.6316, 61.8094) (-17.3812, 62.571) (-18.6779, 62.571) knots 0 0 0 1 2 2 2
  spline S189 degree 2 poles (-18.6779, 62.571) (-19.9541, 62.571) (-21.7449, 61.8094) (-22.4859, 61.0684) knots 0 0 0 1 2 2 2
  spline S190 degree 2 poles (-22.4859, 61.0684) (-23.2063, 60.3068) (-23.9473, 58.4749) (-24.0502, 57.2605) knots 0 0 0 1 2 2 2
  line L146 (-24.0502, 57.2605) -> (-13.9849, 57.2605)
  line L147 (2.5025, 61.2331) -> (2.3378, 61.2331)
  spline S191 degree 2 poles (2.3378, 61.2331) (1.9673, 61.336) (1.1645, 61.3772) (0.6088, 61.3772) knots 0 0 0 1 2 2 2
  spline S192 degree 2 poles (0.6088, 61.3772) (-0.688, 61.3772) (-3.2403, 60.2451) (-4.393, 59.1336) knots 0 0 0 1 2 2 2
  line L148 (-4.393, 59.1336) -> (-4.393, 45.6103)
  line L149 (-4.393, 45.6103) -> (-7.604, 45.6103)
  line L150 (-7.604, 45.6103) -> (-7.604, 64.6705)
  line L151 (-7.604, 64.6705) -> (-4.393, 64.6705)
  line L152 (-4.393, 64.6705) -> (-4.393, 61.83)
  spline S193 degree 2 poles (-4.393, 61.83) (-2.6434, 63.3944) (-0.0293, 64.6705) (1.2057, 64.6705) knots 0 0 0 1 2 2 2
  spline S194 degree 2 poles (1.2057, 64.6705) (1.6997, 64.6705) (2.1937, 64.6294) (2.5025, 64.5676) knots 0 0 0 1 2 2 2
  line L153 (2.5025, 64.5676) -> (2.5025, 61.2331)
  spline S195 degree 2 poles (31.5663, 55.1404) (31.5663, 50.3239) (26.935, 45.0751) (23.0653, 45.0751) knots 0 0 0 1 2 2 2
  spline S196 degree 2 poles (23.0653, 45.0751) (19.0927, 45.0751) (14.5438, 50.4885) (14.5438, 55.1404) knots 0 0 0 1 2 2 2
  spline S197 degree 2 poles (14.5438, 55.1404) (14.5438, 59.9158) (19.2368, 65.2057) (23.0653, 65.2057) knots 0 0 0 1 2 2 2
  spline S198 degree 2 poles (23.0653, 65.2057) (26.935, 65.2057) (31.5663, 59.9363) (31.5663, 55.1404) knots 0 0 0 1 2 2 2
  spline S199 degree 2 poles (28.2524, 55.1404) (28.2524, 58.8454) (25.5559, 62.4475) (23.0653, 62.4475) knots 0 0 0 1 2 2 2
  spline S200 degree 2 poles (23.0653, 62.4475) (20.5747, 62.4475) (17.8577, 58.8454) (17.8577, 55.1404) knots 0 0 0 1 2 2 2
  spline S201 degree 2 poles (17.8577, 55.1404) (17.8577, 51.5383) (20.5747, 47.8333) (23.0653, 47.8333) knots 0 0 0 1 2 2 2
  spline S202 degree 2 poles (23.0653, 47.8333) (25.5354, 47.8333) (28.2524, 51.4765) (28.2524, 55.1404) knots 0 0 0 1 2 2 2
  line L154 (49.8239, 45.6103) -> (46.6128, 45.6103)
  line L155 (46.6128, 45.6103) -> (46.6128, 56.4783)
  spline S203 degree 2 poles (46.6128, 56.4783) (46.6128, 57.7957) (46.3658, 60.0598) (45.9953, 60.7391) knots 0 0 0 1 2 2 2
  spline S204 degree 2 poles (45.9953, 60.7391) (45.6042, 61.4595) (44.2046, 62.1594) (43.0107, 62.1594) knots 0 0 0 1 2 2 2
  spline S205 degree 2 poles (43.0107, 62.1594) (41.8169, 62.1594) (39.2851, 60.8832) (38.0707, 59.854) knots 0 0 0 1 2 2 2
  line L156 (38.0707, 59.854) -> (38.0707, 45.6103)
  line L157 (38.0707, 45.6103) -> (34.8597, 45.6103)
  line L158 (34.8597, 45.6103) -> (34.8597, 64.6705)
  line L159 (34.8597, 64.6705) -> (38.0707, 64.6705)
  line L160 (38.0707, 64.6705) -> (38.0707, 62.5504)
  spline S206 degree 2 poles (38.0707, 62.5504) (39.5115, 63.8472) (42.2903, 65.2057) (43.8547, 65.2057) knots 0 0 0 1 2 2 2
  spline S207 degree 2 poles (43.8547, 65.2057) (46.654, 65.2057) (49.8239, 61.5007) (49.8239, 57.9809) knots 0 0 0 1 2 2 2
  line L161 (49.8239, 57.9809) -> (49.8239, 45.6103)
  spline S208 degree 2 poles (62.6062, 45.178) (58.0367, 45.178) (53.0143, 50.3033) (53.0143, 55.0375) knots 0 0 0 1 2 2 2
  spline S209 degree 2 poles (53.0143, 55.0375) (53.0143, 59.6893) (57.8926, 65.2057) (61.824, 65.2057) knots 0 0 0 1 2 2 2
  spline S210 degree 2 poles (61.824, 65.2057) (63.5942, 65.2057) (66.3318, 64.1765) (67.3404, 63.0856) knots 0 0 0 1 2 2 2
  spline S211 degree 2 poles (67.3404, 63.0856) (68.3696, 61.9947) (69.4605, 58.8454) (69.4605, 56.5607) knots 0 0 0 1 2 2 2
  line L162 (69.4605, 56.5607) -> (69.4605, 54.8111)
  line L163 (69.4605, 54.8111) -> (56.2665, 54.8111)
  spline S212 degree 2 poles (56.2665, 54.8111) (56.2665, 51.4971) (59.601, 47.9774) (62.565, 47.9774) knots 0 0 0 1 2 2 2
  spline S213 degree 2 poles (62.565, 47.9774) (63.6148, 47.9774) (65.6525, 48.4508) (66.4759, 48.8213) knots 0 0 0 1 2 2 2
  spline S214 degree 2 poles (66.4759, 48.8213) (67.3404, 49.2329) (68.5342, 49.9534) (68.9253, 50.2827) knots 0 0 0 1 2 2 2
  line L164 (68.9253, 50.2827) -> (69.1106, 50.2827)
  line L165 (69.1106, 50.2827) -> (69.1106, 46.7835)
  spline S215 degree 2 poles (69.1106, 46.7835) (68.5548, 46.5571) (66.867, 45.8984) (66.2083, 45.7132) knots 0 0 0 1 2 2 2
  spline S216 degree 2 poles (66.2083, 45.7132) (65.282, 45.4456) (63.7589, 45.178) (62.6062, 45.178) knots 0 0 0 1 2 2 2
  spline S217 degree 2 poles (66.3318, 57.2605) (66.2906, 58.5573) (65.7555, 60.4509) (65.2409, 61.089) knots 0 0 0 1 2 2 2
  spline S218 degree 2 poles (65.2409, 61.089) (64.6851, 61.8094) (62.9355, 62.571) (61.6388, 62.571) knots 0 0 0 1 2 2 2
  spline S219 degree 2 poles (61.6388, 62.571) (60.3626, 62.571) (58.5718, 61.8094) (57.8308, 61.0684) knots 0 0 0 1 2 2 2
  spline S220 degree 2 poles (57.8308, 61.0684) (57.1104, 60.3068) (56.3694, 58.4749) (56.2665, 57.2605) knots 0 0 0 1 2 2 2
  line L166 (56.2665, 57.2605) -> (66.3318, 57.2605)
  line L167 (-29.5048, 4.0362) -> (-29.5048, 15.069)
  spline S221 degree 2 poles (-29.5048, 15.069) (-29.5048, 16.3863) (-29.7107, 18.6299) (-30.04, 19.2474) knots 0 0 0 1 2 2 2
  spline S222 degree 2 poles (-30.04, 19.2474) (-30.3693, 19.9267) (-31.6249, 20.5853) (-32.7158, 20.5853) knots 0 0 0 1 2 2 2
  spline S223 degree 2 poles (-32.7158, 20.5853) (-33.7039, 20.5853) (-35.968, 19.3709) (-37.1619, 18.2182) knots 0 0 0 1 2 2 2
  spline S224 degree 2 poles (-37.1619, 18.2182) (-37.1413, 17.9301) (-37.1001, 17.1273) (-37.1001, 16.5921) knots 0 0 0 1 2 2 2
  line L168 (-37.1001, 16.5921) -> (-37.1001, 4.0362)
  line L169 (-37.1001, 4.0362) -> (-40.3111, 4.0362)
  line L170 (-40.3111, 4.0362) -> (-40.3111, 15.069)
  spline S225 degree 2 poles (-40.3111, 15.069) (-40.3111, 16.3863) (-40.517, 18.6299) (-40.8463, 19.2474) knots 0 0 0 1 2 2 2
  spline S226 degree 2 poles (-40.8463, 19.2474) (-41.1757, 19.9267) (-42.4312, 20.5853) (-43.5222, 20.5853) knots 0 0 0 1 2 2 2
  spline S227 degree 2 poles (-43.5222, 20.5853) (-44.5513, 20.5853) (-46.8361, 19.2886) (-47.9064, 18.28) knots 0 0 0 1 2 2 2
  line L171 (-47.9064, 18.28) -> (-47.9064, 4.0362)
  line L172 (-47.9064, 4.0362) -> (-51.1175, 4.0362)
  line L173 (-51.1175, 4.0362) -> (-51.1175, 23.0965)
  line L174 (-51.1175, 23.0965) -> (-47.9064, 23.0965)
  line L175 (-47.9064, 23.0965) -> (-47.9064, 20.997)
  spline S228 degree 2 poles (-47.9064, 20.997) (-46.6509, 22.2526) (-44.1808, 23.6317) (-42.6988, 23.6317) knots 0 0 0 1 2 2 2
  spline S229 degree 2 poles (-42.6988, 23.6317) (-41.011, 23.6317) (-38.3969, 22.0879) (-37.7176, 20.3383) knots 0 0 0 1 2 2 2
  spline S230 degree 2 poles (-37.7176, 20.3383) (-36.2562, 21.9644) (-33.498, 23.6317) (-31.8925, 23.6317) knots 0 0 0 1 2 2 2
  spline S231 degree 2 poles (-31.8925, 23.6317) (-30.6575, 23.6317) (-28.6403, 22.8701) (-27.8993, 22.0056) knots 0 0 0 1 2 2 2
  spline S232 degree 2 poles (-27.8993, 22.0056) (-27.1377, 21.1411) (-26.2938, 18.5476) (-26.2938, 16.5921) knots 0 0 0 1 2 2 2
  line L176 (-26.2938, 16.5921) -> (-26.2938, 4.0362)
  line L177 (-26.2938, 4.0362) -> (-29.5048, 4.0362)
  line L178 (-18.5133, 4.0362) -> (-21.7243, 4.0362)
  line L179 (-21.7243, 4.0362) -> (-21.7243, 23.0965)
  line L180 (-21.7243, 23.0965) -> (-18.5133, 23.0965)
  line L181 (-18.5133, 23.0965) -> (-18.5133, 4.0362)
  line L182 (-18.2868, 26.2664) -> (-21.9301, 26.2664)
  line L183 (-21.9301, 26.2664) -> (-21.9301, 29.6009)
  line L184 (-21.9301, 29.6009) -> (-18.2868, 29.6009)
  line L185 (-18.2868, 29.6009) -> (-18.2868, 26.2664)
  line L186 (1.1645, 4.0362) -> (-2.0465, 4.0362)
  line L187 (-2.0465, 4.0362) -> (-2.0465, 14.9043)
  spline S233 degree 2 poles (-2.0465, 14.9043) (-2.0465, 16.2216) (-2.2935, 18.4858) (-2.664, 19.1651) knots 0 0 0 1 2 2 2
  spline S234 degree 2 poles (-2.664, 19.1651) (-3.0551, 19.8855) (-4.4547, 20.5853) (-5.6486, 20.5853) knots 0 0 0 1 2 2 2
  spline S235 degree 2 poles (-5.6486, 20.5853) (-6.8424, 20.5853) (-9.3742, 19.3092) (-10.5886, 18.28) knots 0 0 0 1 2 2 2
  line L188 (-10.5886, 18.28) -> (-10.5886, 4.0362)
  line L189 (-10.5886, 4.0362) -> (-13.7996, 4.0362)
  line L190 (-13.7996, 4.0362) -> (-13.7996, 23.0965)
  line L191 (-13.7996, 23.0965) -> (-10.5886, 23.0965)
  line L192 (-10.5886, 23.0965) -> (-10.5886, 20.9764)
  spline S236 degree 2 poles (-10.5886, 20.9764) (-9.1478, 22.2732) (-6.369, 23.6317) (-4.8047, 23.6317) knots 0 0 0 1 2 2 2
  spline S237 degree 2 poles (-4.8047, 23.6317) (-2.0053, 23.6317) (1.1645, 19.9267) (1.1645, 16.4069) knots 0 0 0 1 2 2 2
  line L193 (1.1645, 16.4069) -> (1.1645, 4.0362)
  line L194 (20.4924, 4.0362) -> (17.2814, 4.0362)
  line L195 (17.2814, 4.0362) -> (17.2814, 6.1357)
  spline S238 degree 2 poles (17.2814, 6.1357) (15.7994, 4.839) (13.1441, 3.5011) (11.4974, 3.5011) knots 0 0 0 1 2 2 2
  spline S239 degree 2 poles (11.4974, 3.5011) (10.2624, 3.5011) (8.06, 4.3244) (7.2572, 5.2095) knots 0 0 0 1 2 2 2
  spline S240 degree 2 poles (7.2572, 5.2095) (6.4339, 6.0946) (5.5282, 8.791) (5.5282, 10.7259) knots 0 0 0 1 2 2 2
  line L196 (5.5282, 10.7259) -> (5.5282, 23.0965)
  line L197 (5.5282, 23.0965) -> (8.7393, 23.0965)
  line L198 (8.7393, 23.0965) -> (8.7393, 12.2285)
  spline S241 degree 2 poles (8.7393, 12.2285) (8.7393, 10.7053) (8.9657, 8.7087) (9.3568, 7.9677) knots 0 0 0 1 2 2 2
  spline S242 degree 2 poles (9.3568, 7.9677) (9.7478, 7.2267) (11.0858, 6.5474) (12.3414, 6.5474) knots 0 0 0 1 2 2 2
  spline S243 degree 2 poles (12.3414, 6.5474) (13.5146, 6.5474) (16.1699, 7.8853) (17.2814, 8.8528) knots 0 0 0 1 2 2 2
  line L199 (17.2814, 8.8528) -> (17.2814, 23.0965)
  line L200 (17.2814, 23.0965) -> (20.4924, 23.0965)
  line L201 (20.4924, 23.0965) -> (20.4924, 4.0362)
  spline S244 degree 2 poles (30.9076, 3.6657) (28.2935, 3.6657) (25.3501, 6.6503) (25.3501, 9.8819) knots 0 0 0 1 2 2 2
  line L202 (25.3501, 9.8819) -> (25.3501, 20.4413)
  line L203 (25.3501, 20.4413) -> (23.1888, 20.4413)
  line L204 (23.1888, 20.4413) -> (23.1888, 23.0965)
  line L205 (23.1888, 23.0965) -> (25.3501, 23.0965)
  line L206 (25.3501, 23.0965) -> (25.3501, 28.5717)
  line L207 (25.3501, 28.5717) -> (28.5611, 28.5717)
  line L208 (28.5611, 28.5717) -> (28.5611, 23.0965)
  line L209 (28.5611, 23.0965) -> (34.4686, 23.0965)
  line L210 (34.4686, 23.0965) -> (34.4686, 20.4413)
  line L211 (34.4686, 20.4413) -> (28.5611, 20.4413)
  line L212 (28.5611, 20.4413) -> (28.5611, 11.3639)
  spline S245 degree 2 poles (28.5611, 11.3639) (28.5611, 9.9231) (28.6641, 8.3382) (29.014, 7.6589) knots 0 0 0 1 2 2 2
  spline S246 degree 2 poles (29.014, 7.6589) (29.3021, 7.062) (30.5989, 6.4651) (31.7104, 6.4651) knots 0 0 0 1 2 2 2
  spline S247 degree 2 poles (31.7104, 6.4651) (32.4926, 6.4651) (33.954, 6.9385) (34.2833, 7.0826) knots 0 0 0 1 2 2 2
  line L213 (34.2833, 7.0826) -> (34.4686, 7.0826)
  line L214 (34.4686, 7.0826) -> (34.4686, 4.2009)
  spline S248 degree 2 poles (34.4686, 4.2009) (33.5629, 3.9539) (31.7104, 3.6657) (30.9076, 3.6657) knots 0 0 0 1 2 2 2
  spline S249 degree 2 poles (45.1102, 3.604) (40.5407, 3.604) (35.5183, 8.7293) (35.5183, 13.4635) knots 0 0 0 1 2 2 2
  spline S250 degree 2 poles (35.5183, 13.4635) (35.5183, 18.1153) (40.3966, 23.6317) (44.3281, 23.6317) knots 0 0 0 1 2 2 2
  spline S251 degree 2 poles (44.3281, 23.6317) (46.0982, 23.6317) (48.8358, 22.6025) (49.8444, 21.5116) knots 0 0 0 1 2 2 2
  spline S252 degree 2 poles (49.8444, 21.5116) (50.8736, 20.4207) (51.9645, 17.2714) (51.9645, 14.9866) knots 0 0 0 1 2 2 2
  line L215 (51.9645, 14.9866) -> (51.9645, 13.237)
  line L216 (51.9645, 13.237) -> (38.7705, 13.237)
  spline S253 degree 2 poles (38.7705, 13.237) (38.7705, 9.9231) (42.1051, 6.4033) (45.0691, 6.4033) knots 0 0 0 1 2 2 2
  spline S254 degree 2 poles (45.0691, 6.4033) (46.1188, 6.4033) (48.1566, 6.8768) (48.9799, 7.2473) knots 0 0 0 1 2 2 2
  spline S255 degree 2 poles (48.9799, 7.2473) (49.8444, 7.6589) (51.0383, 8.3793) (51.4294, 8.7087) knots 0 0 0 1 2 2 2
  line L217 (51.4294, 8.7087) -> (51.6146, 8.7087)
  line L218 (51.6146, 8.7087) -> (51.6146, 5.2095)
  spline S256 degree 2 poles (51.6146, 5.2095) (51.0589, 4.9831) (49.371, 4.3244) (48.7123, 4.1392) knots 0 0 0 1 2 2 2
  spline S257 degree 2 poles (48.7123, 4.1392) (47.7861, 3.8716) (46.2629, 3.604) (45.1102, 3.604) knots 0 0 0 1 2 2 2
  spline S258 degree 2 poles (48.8358, 15.6865) (48.7947, 16.9832) (48.2595, 18.8769) (47.7449, 19.515) knots 0 0 0 1 2 2 2
  spline S259 degree 2 poles (47.7449, 19.515) (47.1892, 20.2354) (45.4396, 20.997) (44.1428, 20.997) knots 0 0 0 1 2 2 2
  spline S260 degree 2 poles (44.1428, 20.997) (42.8666, 20.997) (41.0759, 20.2354) (40.3349, 19.4944) knots 0 0 0 1 2 2 2
  spline S261 degree 2 poles (40.3349, 19.4944) (39.6145, 18.7328) (38.8735, 16.9009) (38.7705, 15.6865) knots 0 0 0 1 2 2 2
  line L219 (38.7705, 15.6865) -> (48.8358, 15.6865)
  point P0 (0, 0)
  dimension "d6" = 25.4
  constraints: 2 end point, 2 horizontal, 4 other
  measures "d6" distance between parallel lines of L4 L2
emboss "Emboss1" sketch "Sketch3" operation cut depth 2.54 direction (0, 0, -1) wrap yes faces at (42.5763, 135.4667, 70.7231) contours S1 S2 L0 | L0 S2 S3 S4 S5 L5 L6 S6 S7 S8 S9 S10 S11 S12 S13 L7 L8 S14 S15 S0 S1 | L9 L10 L11 L12 L13 L14 L15 L16 | S16 S17 L20 L21 L22 S18 S19 S20 S21 L23 L24 L25 S22 S23 | L26 L27 L28 L29 L30 L31 L32 L33 | L34 L35 L36 L37 L38 L39 L40 L41 L42 L43 L44 L45 | S24 S25 S26 S27 S28 S29 S30 S31 | L46 L47 L48 L49 L50 L51 L52 L53 L54 L55 | S38 S39 S40 S41 S42 S43 L56 L57 S44 S45 S46 S47 S48 S49 L58 L59 L60 L61 L62 S50 S51 | S52 S53 S54 S55 S56 S57 L63 S58 S59 S60 L64 L65 S61 S62 S63 L66 L67 L68 | S68 L70 L71 L72 L73 L74 L75 L76 L77 L78 L79 L80 S69 S70 S71 L81 L82 S72 | S73 S74 S75 S76 L83 L84 S77 S78 S79 L85 L86 S80 S81 | S86 S87 S88 S89 S90 L88 L89 S91 S92 S93 S94 S95 L90 L91 S96 S97 | L92 L93 L94 L95 | S98 S99 S100 S101 | S106 L96 L97 S107 S108 S109 S110 S111 S112 S113 S114 S115 L98 L99 S116 S117 S118 S119 S120 S121 S122 | S123 S124 S125 S126 L100 L101 S127 S128 S129 L102 L103 S130 S131 | S136 L105 L106 S137 S138 S139 S140 S141 S142 S143 S144 S145 L107 L108 S146 S147 S148 S149 S150 S151 S152 | S153 S154 S155 S156 S157 S158 L109 S159 S160 S161 L110 L111 S162 S163 S164 L112 L113 L114 | L116 S169 S170 L117 L118 L119 L120 L121 L122 L123 L124 L125 L126 L127 S171 S172 L128 | S173 L129 L130 L131 L132 L133 L134 L135 L136 L137 L138 L139 S174 S175 S176 L140 L141 S177 | S178 S179 S180 S181 L142 L143 S182 S183 S184 L144 L145 S185 S186 | L147 S191 S192 L148 L149 L150 L151 L152 S193 S194 L153 | S195 S196 S197 S198 | L154 L155 S203 S204 S205 L156 L157 L158 L159 L160 S206 S207 L161 | S208 S209 S210 S211 L162 L163 S212 S213 S214 L164 L165 S215 S216 | L167 S221 S222 S223 S224 L168 L169 L170 S225 S226 S227 L171 L172 L173 L174 L175 S228 S229 S230 S231 S232 L176 L177 | L178 L179 L180 L181 | L182 L183 L184 L185 | L186 L187 S233 S234 S235 L188 L189 L190 L191 L192 S236 S237 L193 | L194 L195 S238 S239 S240 L196 L197 L198 S241 S242 S243 L199 L200 L201 | S244 L202 L203 L204 L205 L206 L207 L208 L209 L210 L211 L212 S245 S246 S247 L213 L214 S248 | S249 S250 S251 S252 L215 L216 S253 S254 S255 L217 L218 S256 S257
body "Solid1"
